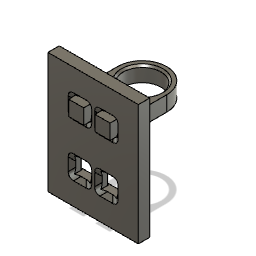
bearing carrier v1 (Autodesk Fusion 360 design; units mm, degrees)
Autodesk Fusion 360 part; units mm, degrees
note: some values were not read from the file. Set by a fixed rule: which sketch regions a step uses.
sketch "Sketch1" plane through (0, 0, 0) normal (0, 1, 0) x (1, 0, 0)
  circle A0 centre (0, 0) radius 5
  circle A1 centre (0, 0) radius 6.5
  line L0 (-6.5, 0) -> (-6.5, -10)
  line L1 (0, -20) -> (0, -2.5)
  line L2 (6.5, 0) -> (6.5, -10)
  line L3 (-6.5, -10) -> (6.5, -10)
  line L4 (-5.5, -10) -> (-5.5, -14)
  line L5 (-5.5, -14) -> (-1.5, -14)
  line L6 (-1.5, -14) -> (-1.5, -10)
  line L7 (0, 0) -> (-6.5, 0) construction
  line L8 (5.5, -10) -> (5.5, -14)
  line L9 (5.5, -14) -> (1.5, -14)
  line L10 (1.5, -14) -> (1.5, -10)
  dimension "d1" = 10
  dimension "d2" = 13
  dimension "d3" = 10
  dimension "d4" = 4
  dimension "d5" = 4
  dimension "d6" = 1
  constraint coincident A0.centre A1.centre
  constraint concentric A0 A1
  constraint coincident A1 L0.start
  constraint vertical L0
  constraint symmetric L0.start L1 L2.start
  constraint symmetric L0.end L1 L2.end
  constraint coincident L3 L4.start
  constraint perpendicular L3 L4
  constraint perpendicular L4 L5
  constraint coincident L3 L6.end
  constraint perpendicular L3 L6
  constraint perpendicular L0 L7
  constraint symmetric L1 L4.start L8.start
  constraint symmetric L1 L4.end L8.end
  constraint symmetric L1 L5.end L9.end
  constraint symmetric L1 L6.end L10.end
  measures "d1" diameter of A0
  measures "d2" diameter of A1
  measures "d3" distance of L0.start L0.end
  measures "d4" distance of L4.start L4.end
  measures "d5" distance of L4.end L5.end
  measures "d6" distance of L0 L4
extrude "Extrude1" add sketch "Sketch1" along normal blind 4 makes body 1
chamfer "Chamfer1" distance 0.5 angle 45 1 edges at (-4.6616, 4, -1.8081) on bodies 1
sketch "Sketch2" plane through (0, 0, 10) normal (0, 0, 1) x (1, 0, 0)
  line L0 (-1.5, 0) -> (1.5, 0)
  line L1 (1.5, 0) -> (1.5, 4)
  line L2 (1.5, 4) -> (-1.5, 4)
  line L3 (-1.5, 4) -> (-1.5, 0)
  line L4 (1.5, 0) -> (5.5, 0)
  line L5 (5.5, 0) -> (5.5, 4)
  line L6 (5.5, 4) -> (1.5, 4)
  line L7 (1.5, 4) -> (1.5, 0)
  line L8 (-5.5, 0) -> (-1.5, 0)
  line L9 (-1.5, 0) -> (-1.5, 4)
  line L10 (-1.5, 4) -> (-5.5, 4)
  line L11 (-5.5, 4) -> (-5.5, 0)
  line L12 (5.6, 4.1) -> (1.4, 4.1)
  line L13 (1.4, 4.1) -> (1.4, -0.1)
  line L14 (1.4, -0.1) -> (5.6, -0.1)
  line L15 (5.6, -0.1) -> (5.6, 4.1)
  line L16 (-1.4, 4.1) -> (-5.6, 4.1)
  line L17 (-5.6, 4.1) -> (-5.6, -0.1)
  line L18 (-5.6, -0.1) -> (-1.4, -0.1)
  line L19 (-1.4, -0.1) -> (-1.4, 4.1)
  line L20 (7.5629, -5) -> (-14.2587, -5) construction
  line L21 (1.4, -9.9) -> (5.6, -9.9)
  line L22 (5.6, -9.9) -> (5.6, -14.1)
  line L23 (5.6, -14.1) -> (1.4, -14.1)
  line L24 (1.4, -14.1) -> (1.4, -9.9)
  line L25 (-1.4, -9.9) -> (-1.4, -14.1)
  line L26 (-5.6, -9.9) -> (-1.4, -9.9)
  line L27 (-5.6, -14.1) -> (-5.6, -9.9)
  line L28 (-1.4, -14.1) -> (-5.6, -14.1)
  line L29 (0, 0) -> (0, -20.6053) construction
  line L30 (-12, 11) -> (12, 11)
  line L31 (12, 11) -> (12, -21)
  line L32 (12, -21) -> (-12, -21)
  line L33 (-12, -21) -> (-12, 11)
  line L34 (-12, 11) -> (12, -21) construction
  line L35 (12, 11) -> (-12, -21) construction
  point P0 (0, -5)
  dimension "d10" = 0.1
  dimension "d11" = 0.1
  dimension "d12" = 5
  dimension "d13" = 24
  dimension "d14" = 32
  constraint horizontal L20
  constraint symmetric L12.start L20 L22.end
  constraint symmetric L12.end L20 L23.end
  constraint symmetric L13.end L20 L21.start
  constraint symmetric L14.end L20 L21.end
  constraint symmetric L16.start L20 L25.end
  constraint symmetric L16.end L20 L27.start
  constraint symmetric L17.end L20 L26.start
  constraint symmetric L18.end L20 L25.start
  constraint coincident L29.start origin
  constraint perpendicular L20 L29
  constraint horizontal L30
  constraint perpendicular L30 L31
  constraint parallel L30 L32
  constraint parallel L31 L33
  constraint coincident L34 P0
  constraint coincident L35 P0
  constraint coincident L29 P0
  constraint coincident L20 P0
  measures "d12" distance of L0 L20
  measures "d13" distance of L31.end L32.end
  measures "d14" distance of L30.end L31.end
extrude "Extrude2" add sketch "Sketch2" along normal blind 3 separate body contours L0 L2 L13 L19 | L30 L31 L32 L33 makes body 2
chamfer "Chamfer2" distance 1 angle 45 16 edges at (3.5, -14.1, 13) (5.6, -12, 13) (3.5, -9.9, 13) (1.4, -12, 13) (-1.4, -12, 13) (-3.5, -14.1, 13) (-5.6, -12, 13) (-3.5, -9.9, 13) (-3.5, -0.1, 13) (-1.4, 2, 13) (-3.5, 4.1, 13) (-5.6, 2, 13) (3.5, -0.1, 13) (5.6, 2, 13) (3.5, 4.1, 13) (1.4, 2, 13) on bodies 2
fillet "Fillet1" radius 2 16 edges at (6.1, -14.6, 12.5) (6.1, -0.6, 12.5) (0.9, -14.6, 12.5) (0.9, -9.4, 12.5) (6.1, -9.4, 12.5) (-0.9, -9.4, 12.5) (-0.9, -14.6, 12.5) (-0.9, -0.6, 12.5) (-6.1, -14.6, 12.5) (-6.1, -9.4, 12.5) (-6.1, -0.6, 12.5) (-6.1, 4.6, 12.5) (-0.9, 4.6, 12.5) (0.9, 4.6, 12.5) (0.9, -0.6, 12.5) (6.1, 4.6, 12.5) on bodies 2
fillet "Fillet2" radius 0.6 8 edges at (-1.4, -12, 10) (-5.6, -12, 10) (5.6, -12, 10) (1.4, -12, 10) (5.6, 2, 10) (1.4, 2, 10) (-1.4, 2, 10) (-5.6, 2, 10) on bodies 2
named bodies: "bearing carrier carrier", "bearing carrier plate"
